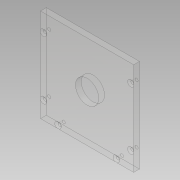
# Autodesk Inventor part: TAPA FRONTAL
Saved by Autodesk Inventor 2019 (Build 230136000, 136)
## iProperties
Created: 2020-04-08
Part Number: TAPA FRONTAL
Material: Plástico PMMA
Document SubType Name: Modeling
Designer: Luis Pujol
Density: 1.188 g/cm^3
Appearance: Policarbonato - Claro
Author: Luis Pujol
Autodesk Inventor part; units mm, degrees
ref_plane "YZ Plane" through (0, 0, 0) normal (1, 0, 0) x (0, 1, 0)
ref_plane "XZ Plane" through (0, 0, 0) normal (0, 1, 0) x (-1, 0, 0)
ref_plane "XY Plane" through (0, 0, 0) normal (0, 0, 1) x (1, 0, 0)
sketch "Boceto1" plane through (0, 0, 0) normal (0, 0, 1) x (1, 0, 0)
  line L0 (-80, -80) -> (80, -80)
  line L1 (80, -80) -> (80, 80)
  line L2 (80, 80) -> (-80, 80)
  line L3 (-80, 80) -> (-80, -80)
  line L4 (-80, -80) -> (80, 80) construction
  line L5 (80, -80) -> (-80, 80) construction
  circle A0 centre (0, 0) radius 20
  dimension "d0" = 160
  dimension "d1" = 160
  dimension "d2" = 40
  constraints: 12 end point, 2 midpoint, 2 parallel, 1 centre point, 1 coincident, 1 horizontal, 1 perpendicular
  measures "d0" distance of L2.end L1.end
  measures "d1" distance of L1.end L0.end
  measures "d2" diameter of A0
extrude "Extrusión1" add sketch "Boceto1" along normal blind 10
sketch "Boceto2" plane through (0, 0, 10) normal (0, 0, 1) x (1, 0, 0)
  line L0 (80, 80) -> (-80, 80) projected
  line L1 (-80, 0) -> (80, 0) construction
  line L2 (80, -80) -> (80, 80) construction
  line L3 (0, -80) -> (0, 80) construction
  line L4 (-80, 80) -> (-80, -80) construction
  line L5 (-80, -80) -> (80, -80) construction
  point P0 (0, 0)
  point P1 (-75, 50)
  point P2 (-75, -50)
  point P3 (75, 50)
  point P4 (75, -50)
  point P5 (-50, -75)
  point P6 (50, -75)
  dimension "d15" = 5
  dimension "d16" = 30
  dimension "d17" = 30
  constraints: 4 end point, 2 midpoint, 2 symmetric about line, 1 horizontal, 1 vertical, 1 other
  measures "d15" distance from line of L4 point (-75, 50)
  measures "d16" distance from line of L0 point (-75, 50)
  measures "d17" distance from line of L5 point (-75, -50)
hole "Agujero1" at (-75, 50, 10) at (-75, -50, 10) at (-50, -75, 10) at (50, -75, 10) at (75, -50, 10) at (75, 50, 10) direction (0, 0, -1) diameter 5.5 depth 20 tip angle 118 countersink diameter 11 countersink angle 90
